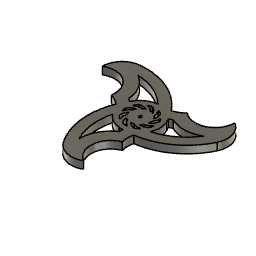
wheel v2 (Autodesk Fusion 360 design; units mm, degrees)
Autodesk Fusion 360 part; units mm, degrees
note: some values were not read from the file. Set by a fixed rule: which sketch regions a step uses.
sketch "스케치1" plane through (0, 0, 0) normal (0, 0, 1) x (1, 0, 0)
  arc A0 (32.8655, -22.8005) -> (32.8655, -77.1995) centre (72.0719, -50) ccw
  arc A1 (32.8655, -22.8005) -> (-32.8655, 22.8005) centre (0, 0) ccw
  arc A2 (-32.8655, 22.8005) -> (-32.8655, -122.8005) centre (72.0719, -50) ccw
  arc A3 (-32.8655, -122.8005) -> (32.8655, -77.1995) centre (0, -100) ccw
  arc A4 (0, 0) -> (0, -100) centre (72.0719, -50) ccw construction
  arc A5 (16.4327, -11.4002) -> (16.4327, -88.5998) centre (72.0719, -50) ccw
  arc A6 (16.4327, -11.4002) -> (-16.4327, 11.4002) centre (0, 0) ccw
  arc A7 (-16.4327, 11.4002) -> (-16.4327, -111.4002) centre (72.0719, -50) ccw
  arc A8 (-16.4327, -111.4002) -> (16.4327, -88.5998) centre (0, -100) ccw
  arc A9 (0, 0) -> (0, -100) centre (72.0719, -50) ccw construction
  circle A10 centre (40, -100) radius 40
  circle A11 centre (40, -100) radius 63.3381
  arc A12 (1.6565, 19.9313) -> (-1.6565, -19.9313) centre (0, 0) ccw
  arc A13 (0, 0) -> (86.6025, 50) centre (7.2653, 87.4161) ccw construction
  arc A14 (3.3131, 39.8626) -> (50.424, 67.0621) centre (7.2653, 87.4161) ccw
  arc A15 (3.3131, 39.8626) -> (-3.3131, -39.8626) centre (0, 0) ccw
  arc A16 (104.6918, 41.469) -> (68.5133, 58.531) centre (86.6025, 50) ccw
  arc A17 (122.7811, 32.9379) -> (50.424, 67.0621) centre (86.6025, 50) ccw
  arc A18 (1.6565, 19.9313) -> (68.5133, 58.531) centre (7.2653, 87.4161) ccw
  arc A19 (-1.6565, -19.9313) -> (104.6918, 41.469) centre (7.2653, 87.4161) ccw
  circle A20 centre (66.6025, 84.641) radius 63.3381
  arc A21 (0, 0) -> (86.6025, 50) centre (7.2653, 87.4161) ccw construction
  arc A22 (-3.3131, -39.8626) -> (122.7811, 32.9379) centre (7.2653, 87.4161) ccw
  circle A23 centre (66.6025, 84.641) radius 40
  arc A24 (-18.0893, -8.531) -> (18.0893, 8.531) centre (0, 0) ccw
  arc A25 (0, 0) -> (-86.6025, 50) centre (-79.3372, -37.4161) ccw construction
  arc A26 (-36.1785, -17.0621) -> (-83.2895, 10.1374) centre (-79.3372, -37.4161) ccw
  arc A27 (-36.1785, -17.0621) -> (36.1785, 17.0621) centre (0, 0) ccw
  arc A28 (-88.2591, 69.9313) -> (-84.946, 30.0687) centre (-86.6025, 50) ccw
  arc A29 (-89.9156, 89.8626) -> (-83.2895, 10.1374) centre (-86.6025, 50) ccw
  arc A30 (-18.0893, -8.531) -> (-84.946, 30.0687) centre (-79.3372, -37.4161) ccw
  arc A31 (18.0893, 8.531) -> (-88.2591, 69.9313) centre (-79.3372, -37.4161) ccw
  circle A32 centre (-106.6025, 15.359) radius 63.3381
  arc A33 (0, 0) -> (-86.6025, 50) centre (-79.3372, -37.4161) ccw construction
  arc A34 (36.1785, 17.0621) -> (-89.9156, 89.8626) centre (-79.3372, -37.4161) ccw
  circle A35 centre (-106.6025, 15.359) radius 40
  dimension "d1" = 100
  dimension "d2" = 80
  dimension "d3" = 40
  dimension "d5" = 360
  constraint tangent A0 A1
  constraint tangent A1 A2
  constraint tangent A2 A3
  constraint tangent A0 A3
  constraint coincident A1.centre A4.start
  constraint tangent A5 A6
  constraint tangent A6 A7
  constraint tangent A7 A8
  constraint tangent A5 A8
  constraint coincident A3.centre A4.end
  constraint coincident A3 A10.centre
  constraint concentric A10 A11
  measures "d1" distance of A3.centre A1.centre
  measures "d2" diameter of A1
  measures "d3" diameter of A6
extrude "돌출1" add sketch "스케치1" along normal blind 30 contours A0 A1 A11 A17 A19 A20 A22 A27 | A1 A5 A19 A27 | A0 A5 A11 A22 A27 | A0 A11 A22 | A0 A11 A22 | A1 A5 A6 A18 A19 A24 A27 A31 | A5 A7 A12 A15 A19 A24 A27 A30 | A5 A22 A27 | A0 A5 A10 A11 A22 | A5 A11 A22 | A1 A18 A34 | A5 A19 A24 | A16 A18 A19 A20 A23 | A16 A17 A19 A20 A23 | A5 A7 A8 A10 A11 | A1 A15 A18 A31 | A1 A14 A18 A20 A34 | A18 A20 A34 | A6 A12 A24 | A14 A18 A20 A23 A34 | A7 A15 A27 A30 | A2 A3 A7 A11 A15 A26 A27 A32 | A3 A7 A8 A10 A11 | A1 A14 A15 A20 A29 A31 A32 A34 | A6 A18 A31 | A1 A6 A7 A12 A15 A18 A30 A31 | A14 A20 A34 | A7 A12 A30 | A2 A15 A26 A30 A32 | A14 A20 A34 | A2 A15 A30 | A2 A26 A32 | A2 A26 A32 | A28 A30 A31 A32 A35 | A28 A29 A31 A32 A35 | A2 A30 A32 | A2 A26 A30 A32 A35
sketch "스케치2" plane through (0, 0, 30) normal (0, 0, 1) x (-1, 0, 0)
  arc A0 (-36.5535, 16.2433) -> (-98.2716, -29.7887) centre (-7.2653, -87.4161) ccw
  arc A1 (-36.5535, 16.2433) -> (-36.1785, -17.0621) centre (0, 0) ccw
  arc A2 (-36.1785, -17.0621) -> (-32.3578, -24.5192) centre (79.3372, 37.4161) ccw
  arc A3 (-32.3578, -24.5192) -> (-39.0384, -27.6153) centre (-7.2653, -87.4161) ccw
  arc A4 (-39.0384, -27.6153) -> (-98.2716, -29.7887) centre (-66.6025, -84.641) ccw
  arc A5 (32.3438, 23.5346) -> (3.3131, 39.8626) centre (0, 0) ccw
  arc A6 (3.3131, 39.8626) -> (-5.0553, 40.2823) centre (-7.2653, -87.4161) ccw
  arc A7 (-5.0553, 40.2823) -> (-4.3964, 47.6159) centre (-72.0719, 50) ccw
  arc A8 (-4.3964, 47.6159) -> (23.3381, 100) centre (-40, 100) ccw
  arc A9 (32.3438, 23.5346) -> (23.3381, 100) centre (-72.0719, 50) ccw
  arc A10 (4.2097, -39.7779) -> (74.9335, -70.2113) centre (79.3372, 37.4161) ccw
  arc A11 (4.2097, -39.7779) -> (32.8655, -22.8005) centre (0, 0) ccw
  arc A12 (32.8655, -22.8005) -> (37.4131, -15.7631) centre (-72.0719, 50) ccw
  arc A13 (37.4131, -15.7631) -> (43.4348, -20.0006) centre (79.3372, 37.4161) ccw
  arc A14 (43.4348, -20.0006) -> (74.9335, -70.2113) centre (106.6025, -15.359) ccw
  arc A15 (46.5737, 2.7244) -> (32.8655, 122.8005) centre (-72.0719, 50) ccw
  arc A16 (32.8655, 122.8005) -> (-20, 134.641) centre (0, 100) ccw
  arc A17 (-26.0262, 62.5202) -> (-20, 134.641) centre (-40, 100) ccw
  arc A18 (-25.6463, 38.9718) -> (-26.0262, 62.5202) centre (-72.0719, 50) ccw
  arc A19 (-25.6463, 38.9718) -> (-122.7811, -32.9379) centre (-7.2653, -87.4161) ccw
  arc A20 (-122.7811, -32.9379) -> (-106.6025, -84.641) centre (-86.6025, -50) ccw
  arc A21 (-41.131, -53.7995) -> (-106.6025, -84.641) centre (-66.6025, -84.641) ccw
  arc A22 (-20.9274, -41.6962) -> (-41.131, -53.7995) centre (-7.2653, -87.4161) ccw
  arc A23 (-20.9274, -41.6962) -> (89.9156, -89.8626) centre (79.3372, 37.4161) ccw
  arc A24 (89.9156, -89.8626) -> (126.6025, -50) centre (86.6025, -50) ccw
  arc A25 (67.1572, -8.7207) -> (126.6025, -50) centre (106.6025, -15.359) ccw
  arc A26 (46.5737, 2.7244) -> (67.1572, -8.7207) centre (79.3372, 37.4161) ccw
  circle A27 centre (0, 0) radius 30
  circle A28 centre (0, 0) radius 20
  arc A29 (0.9818, -2.2991) -> (0.9818, 32.2991) centre (-6.4058, 15) ccw
  arc A30 (-0.9818, 2.2991) -> (0.9818, -2.2991) centre (0, 0) ccw
  arc A31 (-0.9818, 2.2991) -> (-0.9818, 27.7009) centre (-6.4058, 15) ccw
  arc A32 (0.9818, 32.2991) -> (-0.9818, 27.7009) centre (0, 30) ccw
  arc A33 (0, 0) -> (0, 30) centre (-6.4058, 15) ccw construction
  arc A34 (-2.23, 1.1301) -> (-18.5579, 20.589) centre (-14.5489, 7.3731) ccw
  arc A35 (2.23, -1.1301) -> (-20.0093, 25.3737) centre (-14.5489, 7.3731) ccw
  arc A36 (-20.0093, 25.3737) -> (-18.5579, 20.589) centre (-19.2836, 22.9813) ccw
  arc A37 (-2.23, 1.1301) -> (2.23, -1.1301) centre (0, 0) ccw
  arc A38 (-2.4347, -0.5677) -> (-27.4505, 3.8433) centre (-15.8845, -3.7037) ccw
  arc A39 (2.4347, 0.5677) -> (-31.6379, 6.5756) centre (-15.8845, -3.7037) ccw
  arc A40 (-31.6379, 6.5756) -> (-27.4505, 3.8433) centre (-29.5442, 5.2094) ccw
  arc A41 (-2.4347, -0.5677) -> (2.4347, 0.5677) centre (0, 0) ccw
  arc A42 (-1.5002, -1.9999) -> (-23.4987, -14.7007) centre (-9.7875, -13.0476) ccw
  arc A43 (1.5002, 1.9999) -> (-28.4628, -15.2993) centre (-9.7875, -13.0476) ccw
  arc A44 (-28.4628, -15.2993) -> (-23.4987, -14.7007) centre (-25.9808, -15) ccw
  arc A45 (-1.5002, -1.9999) -> (1.5002, 1.9999) centre (0, 0) ccw
  arc A46 (0.1363, -2.4963) -> (-8.5516, -26.3661) centre (0.8892, -16.2863) ccw
  arc A47 (-0.1363, 2.4963) -> (-11.9696, -30.0154) centre (0.8892, -16.2863) ccw
  arc A48 (-11.9696, -30.0154) -> (-8.5516, -26.3661) centre (-10.2606, -28.1908) ccw
  arc A49 (0.1363, -2.4963) -> (-0.1363, 2.4963) centre (0, 0) ccw
  arc A50 (1.709, -1.8247) -> (10.3969, -25.6945) centre (11.1498, -11.9045) ccw
  arc A51 (-1.709, 1.8247) -> (10.1243, -30.6871) centre (11.1498, -11.9045) ccw
  arc A52 (10.1243, -30.6871) -> (10.3969, -25.6945) centre (10.2606, -28.1908) ccw
  arc A53 (1.709, -1.8247) -> (-1.709, 1.8247) centre (0, 0) ccw
  arc A54 (2.482, -0.2993) -> (24.4806, -13.0001) centre (16.1933, -1.9524) ccw
  arc A55 (-2.482, 0.2993) -> (27.4809, -16.9999) centre (16.1933, -1.9524) ccw
  arc A56 (27.4809, -16.9999) -> (24.4806, -13.0001) centre (25.9808, -15) ccw
  arc A57 (2.482, -0.2993) -> (-2.482, 0.2993) centre (0, 0) ccw
  arc A58 (2.0937, 1.3662) -> (27.1095, 5.7771) centre (13.6598, 8.9132) ccw
  arc A59 (-2.0937, -1.3662) -> (31.9789, 4.6418) centre (13.6598, 8.9132) ccw
  arc A60 (31.9789, 4.6418) -> (27.1095, 5.7771) centre (29.5442, 5.2094) ccw
  arc A61 (2.0937, 1.3662) -> (-2.0937, -1.3662) centre (0, 0) ccw
  arc A62 (0.7257, 2.3924) -> (17.0536, 21.8512) centre (4.7347, 15.6082) ccw
  arc A63 (-0.7257, -2.3924) -> (21.5136, 24.1114) centre (4.7347, 15.6082) ccw
  arc A64 (21.5136, 24.1114) -> (17.0536, 21.8512) centre (19.2836, 22.9813) ccw
  arc A65 (0.7257, 2.3924) -> (-0.7257, -2.3924) centre (0, 0) ccw
  dimension "d8" = 60
  dimension "d9" = 40
  dimension "d10" = 5
  dimension "d12" = 360
  constraint concentric A1 A27
  constraint concentric A1 A28
  constraint tangent A29 A30
  constraint tangent A30 A31
  constraint tangent A31 A32
  constraint tangent A29 A32
  constraint coincident A1.centre A5.centre
  constraint coincident A27 A32.centre
  measures "d8" diameter of A27
  measures "d9" diameter of A28
  measures "d10" diameter of A32
extrude "돌출2" cut sketch "스케치2" against normal blind 30 contours A27 A28 A58 A59 A60 | A27 A28 A62 A63 A64 | A27 A28 A54 A55 A56 | A27 A28 A29 A31 A32 | A27 A28 A50 A51 A52 | A27 A28 A34 A35 A36 | A27 A28 A46 A47 A48 | A27 A28 A38 A39 A40 | A27 A28 A42 A43 A44
sketch "스케치3" plane through (0, 0, 30) normal (0, 0, 1) x (-1, 0, 0)
  arc A0 (4.805, -29.6127) -> (12.5722, -27.2386) centre (0, 0) ccw
  arc A1 (-6.2753, -18.99) -> (4.805, -29.6127) centre (11.1498, -11.9045) ccw
  arc A2 (-6.2753, -18.99) -> (-0.0393, -20) centre (0, 0) ccw
  arc A3 (-0.0393, -20) -> (10.3969, -25.6945) centre (11.1498, -11.9045) ccw
  arc A4 (12.5722, -27.2386) -> (10.3969, -25.6945) centre (10.2606, -28.1908) ccw
  arc A5 (5.6129, 29.4702) -> (-2.4978, 29.8958) centre (0, 0) ccw
  arc A6 (12.3918, 15.6985) -> (5.6129, 29.4702) centre (-6.4058, 15) ccw
  arc A7 (12.3918, 15.6985) -> (6.8773, 18.7804) centre (0, 0) ccw
  arc A8 (6.8773, 18.7804) -> (-0.9818, 27.7009) centre (-6.4058, 15) ccw
  arc A9 (-2.4978, 29.8958) -> (-0.9818, 27.7009) centre (0, 30) ccw
  arc A10 (-14.6434, 26.1834) -> (-21.1301, 21.296) centre (0, 0) ccw
  arc A11 (-0.5981, 19.9911) -> (-14.6434, 26.1834) centre (-14.5489, 7.3731) ccw
  arc A12 (-0.5981, 19.9911) -> (-6.8035, 18.8072) centre (0, 0) ccw
  arc A13 (-6.8035, 18.8072) -> (-18.5579, 20.589) centre (-14.5489, 7.3731) ccw
  arc A14 (-21.1301, 21.296) -> (-18.5579, 20.589) centre (-19.2836, 22.9813) ccw
  arc A15 (22.7155, -19.596) -> (27.1395, -12.7847) centre (0, 0) ccw
  arc A16 (7.3994, -18.5809) -> (22.7155, -19.596) centre (16.1933, -1.9524) ccw
  arc A17 (7.3994, -18.5809) -> (12.8256, -15.3461) centre (0, 0) ccw
  arc A18 (12.8256, -15.3461) -> (24.4806, -13.0001) centre (16.1933, -1.9524) ccw
  arc A19 (27.1395, -12.7847) -> (24.4806, -13.0001) centre (25.9808, -15) ccw
  arc A20 (-15.3538, -25.7732) -> (-7.8778, -28.9472) centre (0, 0) ccw
  arc A21 (-17.0137, -10.5135) -> (-15.3538, -25.7732) centre (0.8892, -16.2863) ccw
  arc A22 (-17.0137, -10.5135) -> (-12.8858, -15.2956) centre (0, 0) ccw
  arc A23 (-12.8858, -15.2956) -> (-8.5516, -26.3661) centre (0.8892, -16.2863) ccw
  arc A24 (-7.8778, -28.9472) -> (-8.5516, -26.3661) centre (-10.2606, -28.1908) ccw
  arc A25 (23.2428, 18.9676) -> (17.3032, 24.5071) centre (0, 0) ccw
  arc A26 (19.5835, 4.0605) -> (23.2428, 18.9676) centre (4.7347, 15.6082) ccw
  arc A27 (19.5835, 4.0605) -> (17.3401, 9.966) centre (0, 0) ccw
  arc A28 (17.3401, 9.966) -> (17.0536, 21.8512) centre (4.7347, 15.6082) ccw
  arc A29 (17.3032, 24.5071) -> (17.0536, 21.8512) centre (19.2836, 22.9813) ccw
  arc A30 (-28.0479, 10.6451) -> (-29.8754, 2.7315) centre (0, 0) ccw
  arc A31 (-13.3082, 14.9296) -> (-28.0479, 10.6451) centre (-15.8845, -3.7037) ccw
  arc A32 (-13.3082, 14.9296) -> (-17.3008, 10.034) centre (0, 0) ccw
  arc A33 (-17.3008, 10.034) -> (-27.4505, 3.8433) centre (-15.8845, -3.7037) ccw
  arc A34 (-29.8754, 2.7315) -> (-27.4505, 3.8433) centre (-29.5442, 5.2094) ccw
  arc A35 (29.9972, -0.4102) -> (29.0079, 7.6512) centre (0, 0) ccw
  arc A36 (17.6118, -9.4775) -> (29.9972, -0.4102) centre (13.6598, 8.9132) ccw
  arc A37 (17.6118, -9.4775) -> (19.6893, -3.5116) centre (0, 0) ccw
  arc A38 (19.6893, -3.5116) -> (27.1095, 5.7771) centre (13.6598, 8.9132) ccw
  arc A39 (29.0079, 7.6512) -> (27.1095, 5.7771) centre (29.5442, 5.2094) ccw
  arc A40 (-28.3284, -9.8742) -> (-24.6416, -17.1111) centre (0, 0) ccw
  arc A41 (-19.7912, 2.8823) -> (-28.3284, -9.8742) centre (-9.7875, -13.0476) ccw
  arc A42 (-19.7912, 2.8823) -> (-19.7029, -3.4343) centre (0, 0) ccw
  arc A43 (-19.7029, -3.4343) -> (-23.4987, -14.7007) centre (-9.7875, -13.0476) ccw
  arc A44 (-24.6416, -17.1111) -> (-23.4987, -14.7007) centre (-25.9808, -15) ccw
  arc A45 (-36.5535, 16.2433) -> (-98.2716, -29.7887) centre (-7.2653, -87.4161) ccw
  arc A46 (-36.5535, 16.2433) -> (-36.1785, -17.0621) centre (0, 0) ccw
  arc A47 (-36.1785, -17.0621) -> (-32.3578, -24.5192) centre (79.3372, 37.4161) ccw
  arc A48 (-32.3578, -24.5192) -> (-39.0384, -27.6153) centre (-7.2653, -87.4161) ccw
  arc A49 (-39.0384, -27.6153) -> (-98.2716, -29.7887) centre (-66.6025, -84.641) ccw
  arc A50 (32.3438, 23.5346) -> (3.3131, 39.8626) centre (0, 0) ccw
  arc A51 (3.3131, 39.8626) -> (-5.0553, 40.2823) centre (-7.2653, -87.4161) ccw
  arc A52 (-5.0553, 40.2823) -> (-4.3964, 47.6159) centre (-72.0719, 50) ccw
  arc A53 (-4.3964, 47.6159) -> (23.3381, 100) centre (-40, 100) ccw
  arc A54 (32.3438, 23.5346) -> (23.3381, 100) centre (-72.0719, 50) ccw
  arc A55 (4.2097, -39.7779) -> (74.9335, -70.2113) centre (79.3372, 37.4161) ccw
  arc A56 (4.2097, -39.7779) -> (32.8655, -22.8005) centre (0, 0) ccw
  arc A57 (32.8655, -22.8005) -> (37.4131, -15.7631) centre (-72.0719, 50) ccw
  arc A58 (37.4131, -15.7631) -> (43.4348, -20.0006) centre (79.3372, 37.4161) ccw
  arc A59 (43.4348, -20.0006) -> (74.9335, -70.2113) centre (106.6025, -15.359) ccw
  arc A60 (46.5737, 2.7244) -> (32.8655, 122.8005) centre (-72.0719, 50) ccw
  arc A61 (32.8655, 122.8005) -> (-20, 134.641) centre (0, 100) ccw
  arc A62 (-26.0262, 62.5202) -> (-20, 134.641) centre (-40, 100) ccw
  arc A63 (-25.6463, 38.9718) -> (-26.0262, 62.5202) centre (-72.0719, 50) ccw
  arc A64 (-25.6463, 38.9718) -> (-122.7811, -32.9379) centre (-7.2653, -87.4161) ccw
  arc A65 (-122.7811, -32.9379) -> (-106.6025, -84.641) centre (-86.6025, -50) ccw
  arc A66 (-41.131, -53.7995) -> (-106.6025, -84.641) centre (-66.6025, -84.641) ccw
  arc A67 (-20.9274, -41.6962) -> (-41.131, -53.7995) centre (-7.2653, -87.4161) ccw
  arc A68 (-20.9274, -41.6962) -> (89.9156, -89.8626) centre (79.3372, 37.4161) ccw
  arc A69 (89.9156, -89.8626) -> (126.6025, -50) centre (86.6025, -50) ccw
  arc A70 (67.1572, -8.7207) -> (126.6025, -50) centre (106.6025, -15.359) ccw
  arc A71 (46.5737, 2.7244) -> (67.1572, -8.7207) centre (79.3372, 37.4161) ccw
  circle A72 centre (0, 0) radius 2.75
  line L0 (-2.75, 0) -> (1.95, 0)
  line L1 (1.95, 0) -> (1.95, -1.9391)
  line L2 (1.95, 0) -> (1.95, 1.9391)
  dimension "d15" = 5.5
  dimension "d16" = 4.7
  constraint coincident A0.centre A2.centre
  constraint coincident A72 L0.start
  constraint horizontal L0
  constraint coincident A72 L1.end
  constraint perpendicular L0 L1
  constraint coincident A72 L2.end
  constraint perpendicular L0 L2
  measures "d15" diameter of A72
  measures "d16" distance of L0.start L0.end
extrude "돌출3" cut sketch "스케치3" against normal blind 30 contours A72 L0 L2 | A72 L0 L1
extrude "돌출4" cut 1 faces at (-16.7209, -113.5942, 30) along direction (0, 0, -1) blind 15
